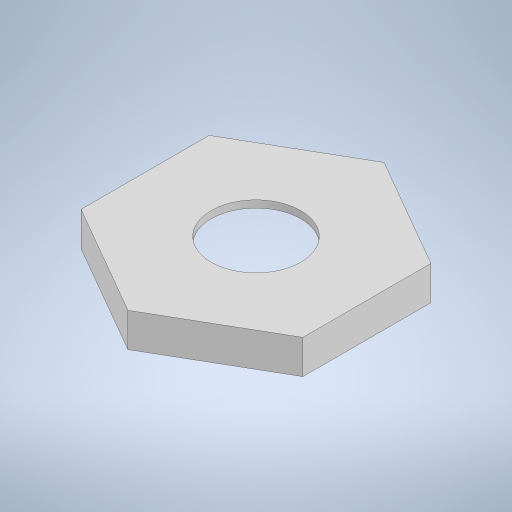
# Autodesk Inventor part: держатель
Saved by Autodesk Inventor 2024 (Build 280153000, 153)
## iProperties
Created: 2025-08-14
Part Number: держатель
Material: Типовые
Document SubType Name: Modeling
Designer: DELL
Density: 1 g/cm^3
Appearance: По умолчанию
Author: DELL
Autodesk Inventor part; units mm, degrees
ref_plane "YZ Plane" through (0, 0, 0) normal (1, 0, 0) x (0, 1, 0)
ref_plane "XZ Plane" through (0, 0, 0) normal (0, 1, 0) x (-1, 0, 0)
ref_plane "XY Plane" through (0, 0, 0) normal (0, 0, 1) x (1, 0, 0)
sketch "Эскиз1" plane through (0, 0, 0) normal (0, 1, 0) x (-1, 0, 0)
  line L0 (-23, 13.2791) -> (0, 26.5581)
  line L1 (0, 26.5581) -> (23, 13.2791)
  line L2 (23, 13.2791) -> (23, -13.2791)
  line L3 (23, -13.2791) -> (0, -26.5581)
  line L4 (0, -26.5581) -> (-23, -13.2791)
  line L5 (-23, -13.2791) -> (-23, 13.2791)
  line L6 (0, 0) -> (15.979, 0)
  line L7 (0, 0) -> (15.979, 0) construction
  line L8 (31, -17.8979) -> (31, 17.8979)
  line L9 (31, 17.8979) -> (0, 35.7957)
  line L10 (0, 35.7957) -> (-31, 17.8979)
  line L11 (-31, 17.8979) -> (-31, -17.8979)
  line L12 (-31, -17.8979) -> (0, -35.7957)
  line L13 (0, -35.7957) -> (31, -17.8979)
  dimension "d2" = 46
  dimension "d3" = 8
  constraints: 28 end point, 2 horizontal, 1 coincident, 1 collinear, 1 perpendicular, 18 other
  measures "d2" distance between parallel lines of L1 L4
  measures "d3" distance between parallel lines of L2 L8
extrude "Выдавливание1" add sketch "Эскиз1" along normal blind 7.5
sketch "Эскиз2" plane through (0, 7.5, 0) normal (0, 1, 0) x (1, 0, 0)
  line L0 (31, -17.8979) -> (31, 17.8979) projected
  line L1 (31, 17.8979) -> (31, -17.8979)
  line L2 (31, -17.8979) -> (0, -35.7957)
  line L3 (0, -35.7957) -> (-31, -17.8979)
  line L4 (-31, -17.8979) -> (-31, 17.8979)
  line L5 (-31, 17.8979) -> (0, 35.7957)
  line L6 (0, 35.7957) -> (31, 17.8979)
  circle A0 centre (0, 0) radius 12.5
  point P0 (31, -17.8979)
  dimension "d6" = 25
  constraints: 12 end point, 2 coincident, 1 centre point, 13 other
  measures "d6" diameter of A0
extrude "Выдавливание2" add sketch "Эскиз2" along normal blind 2
sketch "Эскиз3" plane through (0, 0, 0) normal (0, -1, 0) x (1, 0, 0)
  line L0 (0, 35.7957) -> (31, 17.8979) construction
  line L1 (15.5, 26.8468) -> (11.5, 19.9186) construction
  line L2 (23, 13.2791) -> (0, 26.5581) construction
  circle A0 centre (13.5, 23.3827) radius 2
  circle A1 centre (0, 0) radius 27 construction
  circle A2 centre (-13.5, 23.3827) radius 2
  circle A3 centre (-27, 0) radius 2
  circle A4 centre (-13.5, -23.3827) radius 2
  circle A5 centre (13.5, -23.3827) radius 2
  circle A6 centre (27, 0) radius 2
  dimension "d9" = 4
  dimension "d12" = 360
  constraints: 6 centre point, 3 midpoint, 2 end point, 1 coincident, 16 other
  measures "d9" diameter of A0
extrude "Выдавливание3" cut sketch "Эскиз3" against normal blind 4
